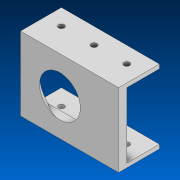
# Autodesk Inventor part: Inner Channel Guide
Saved by Autodesk Inventor 2022.2 (Build 262287000, 287)
## iProperties
Created: 2022-03-25
Part Number: Inner Channel Guide
Material: Generic
Document SubType Name: Modeling
Designer: omard
Density: 1 g/cm^3
Appearance: Default
Author: omard
Autodesk Inventor part; units mm, degrees
ref_plane "YZ Plane" through (0, 0, 0) normal (1, 0, 0) x (0, 1, 0)
ref_plane "XZ Plane" through (0, 0, 0) normal (0, 1, 0) x (-1, 0, 0)
ref_plane "XY Plane" through (0, 0, 0) normal (0, 0, 1) x (1, 0, 0)
sketch "Sketch1" plane through (0, 0, 0) normal (0, 0, 1) x (1, 0, 0)
  circle A0 centre (0, 0) radius 15.875
  line L0 (0, 15.875) -> (0, 25.4)
  line L1 (0, 25.4) -> (-30.5689, 25.4)
  line L2 (-30.5689, 25.4) -> (-30.5689, -25.4)
  line L3 (-30.5689, -25.4) -> (0, -25.4)
  line L4 (0, -25.4) -> (0, -15.875)
  line L5 (0, -15.875) -> (0, 15.875)
  line L6 (0, 25.4) -> (45.6311, 25.4)
  line L7 (45.6311, 25.4) -> (45.6311, -25.4)
  line L8 (45.6311, -25.4) -> (0, -25.4)
  line L9 (0, -25.4) -> (0, 25.4)
  line L10 (7.5311, 25.4) -> (7.5311, -25.4) construction
  line L11 (-17.8689, 25.4) -> (-17.8689, -25.4) construction
  line L12 (32.9311, 25.4) -> (32.9311, -25.4) construction
  dimension "d0" = 31.75
  dimension "d1" = 50.8
  dimension "d3" = 7.5311
  dimension "d6" = 38.1
  dimension "d7" = 38.1
  dimension "d8" = 25.4
  dimension "d9" = 25.4
  constraints: 26 end point, 8 point on line, 6 perpendicular, 3 vertical, 2 collinear, 2 parallel, 2 point on circle, 1 centre point, 1 coincident, 1 horizontal, 1 vertical alignment
  measures "d0" diameter of A0
  measures "d1" distance between parallel lines of L3 L1
  measures "d3" distance between parallel lines of L0 L10
  measures "d6" distance between parallel lines of L10 L2
  measures "d7" distance between parallel lines of L7 L10
  measures "d8" distance between parallel lines of L10 L11
  measures "d9" distance between parallel lines of L12 L10
extrude "Extrusion1" add sketch "Sketch1" along normal blind 6.35 contours A0 L0 L6 L7 L8 L4 | A0 L4 L3 L2 L1 L0
chamfer "Chamfer1" distance 6.35 distance2 6.35 1 edges at (-15.875, 0, 0) measured on face at (-15.875, 0, 0.5)
sketch "Sketch2" plane through (-30.5689, -25.4, 0) normal (-1, 0, 0) x (0, 0, 1)
  line L0 (0, 0) -> (6.35, 0) projected
  line L1 (6.35, 0) -> (-25.4, 0)
  line L2 (-25.4, 0) -> (-25.4, -3.175)
  line L3 (-25.4, -3.175) -> (6.35, -3.175)
  line L4 (6.35, -3.175) -> (6.35, 0)
  line L5 (6.35, 50.8) -> (-25.4, 50.8)
  line L6 (-25.4, 50.8) -> (-25.4, 53.975)
  line L7 (-25.4, 53.975) -> (6.35, 53.975)
  line L8 (6.35, 53.975) -> (6.35, 50.8)
  line L9 (0, 50.8) -> (0, 0) projected
  point P0 (0, 25.4)
  dimension "d15" = 3.175
  dimension "d16" = 25.4
  constraints: 16 end point, 4 parallel, 2 equal length, 2 horizontal, 2 perpendicular
  measures "d15" distance between parallel lines of L1 L3
  measures "d16" distance between parallel lines of L9 L2
extrude "Extrusion2" add sketch "Sketch2" against normal up to surface (76.2 mm away)
sketch "Sketch3" plane through (-30.5689, 28.575, 6.35) normal (0, 1, 0) x (1, 0, 0)
  line L0 (0, 0) -> (0, 31.75) projected
  line L1 (0, 31.75) -> (76.2, 31.75) projected
  point P0 (30.5689, 6.35)
  point P1 (12.7, 19.05)
  point P2 (38.1, 19.05)
  point P3 (63.5, 19.05)
  dimension "d19" = 12.7
  dimension "d20" = 25.4
  dimension "d21" = 25.4
  dimension "d22" = 12.7
  constraints: 2 horizontal alignment
  measures "d19" distance from line of L0 point (12.7, 19.05)
  measures "d20" distance of point (12.7, 19.05) point (38.1, 19.05)
  measures "d21" distance of point (38.1, 19.05) point (63.5, 19.05)
  measures "d22" distance from line of L1 point (12.7, 19.05)
hole "Hole1" at (-17.8689, 28.575, -12.7) at (7.5311, 28.575, -12.7) at (32.9311, 28.575, -12.7) direction (0, -1, 0) diameter 4.445 end through all start extended yes
sketch "Sketch4" plane through (0, 0, 0) normal (0, 0, -1) x (-1, 0, 0)
  line L0 (22.225, -15.875) -> (-22.225, -15.875)
  line L1 (-22.225, -15.875) -> (-22.225, 15.875)
  line L2 (-22.225, 15.875) -> (22.225, 15.875)
  line L3 (22.225, 15.875) -> (22.225, -15.875)
  line L4 (22.225, -15.875) -> (-22.225, 15.875) construction
  line L5 (-22.225, -15.875) -> (22.225, 15.875) construction
  circle A0 centre (0, 0) radius 15.875 projected
  circle A1 centre (0, 0) radius 22.225 projected
  point P0 (15.5543, 15.875)
  point P1 (-15.5543, 15.875)
  point P2 (-15.5543, -15.875)
  point P3 (15.5543, -15.875)
  constraints: 12 end point, 2 midpoint, 2 parallel, 2 tangent, 1 horizontal, 1 perpendicular
extrude "Extrusion3" add sketch "Sketch4" against normal up to surface (6.35 mm away) contours A1 L0 | L2 A1
body "Solid1"
